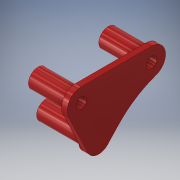
# Autodesk Inventor part: Idle pulley pin
Saved by Autodesk Inventor 2019.4 (Build 234330000, 330)
## iProperties
Created: 2020-02-23
Part Number: Idle pulley pin
Material: ABS Plastic
Document SubType Name: Modeling
Designer: admin
Density: 1.06 g/cm^3
Appearance: Red
Author: admin
Autodesk Inventor part; units mm, degrees
ref_plane "YZ Plane" through (0, 0, 0) normal (1, 0, 0) x (0, 1, 0)
ref_plane "XZ Plane" through (0, 0, 0) normal (0, 1, 0) x (-1, 0, 0)
ref_plane "XY Plane" through (0, 0, 0) normal (0, 0, 1) x (1, 0, 0)
sketch "Sketch3" plane through (0, 0, 0) normal (1, 0, 0) x (0, 1, 0)
  circle A0 centre (21.8648, -65.6605) radius 2.75 projected
  circle A1 centre (21.8648, -28.1605) radius 2.75 projected
  circle A2 centre (21.8648, 9.3395) radius 2.75 projected
  line L0 (21.8648, -65.6605) -> (21.8648, 9.3395) construction
  line L1 (29.3648, -65.6605) -> (29.3648, -28.1605) construction
  line L2 (14.3648, 9.3395) -> (14.3648, -22.1411) construction
  arc A3 (14.3648, -65.6605) -> (29.3648, -65.6605) centre (21.8648, -65.6605) ccw construction
  arc A4 (29.3648, 9.3395) -> (18.6312, 16.1066) centre (21.8648, 9.3395) ccw
  circle A5 centre (0, 0) radius 6.5
  line L3 (-2.8024, 5.8648) -> (18.6312, 16.1066)
  line L4 (-4.4137, -4.7717) -> (14.3648, -22.1411)
  arc A6 (18.6312, 16.1066) -> (14.3648, 9.3395) centre (21.8648, 9.3395) ccw
  line L5 (14.3648, -22.1411) -> (14.3648, -28.1605)
  circle A7 centre (21.8648, -28.1605) radius 7.5
  line L6 (29.3648, -28.1605) -> (29.3648, 9.3395)
  line L7 (14.3648, -28.1605) -> (14.3648, -65.6605) construction
  dimension "d14" = 15
  dimension "d15" = 13
  constraints: 21 tangent, 18 end point, 10 point on circle, 6 parallel, 5 centre point, 2 coincident, 1 midpoint, 1 vertical
  measures "d14" diameter of A4
  measures "d15" diameter of A5
extrude "Extrusion2" add sketch "Sketch3" along normal blind 3 contours L6 A7 L5 L4 A5 L3 A4 | A7 | A5
sketch "Sketch4" plane through (0, 0, 0) normal (-1, 0, 0) x (0, 0, 1)
  arc A0 (-4.7717, -4.4137) -> (5.8648, -2.8024) centre (0, 0) ccw projected
  circle A1 centre (0, 0) radius 5
  dimension "d18" = 10
  constraints: 1 centre point, 1 coincident
  measures "d18" diameter of A1
extrude "Extrusion3" add sketch "Sketch4" along normal blind 25.1
sketch "Sketch5" plane through (0, 0, 0) normal (1, 0, 0) x (0, 0, -1)
  circle A0 centre (0, 0) radius 6.5
  dimension "d23" = 13
  constraints: 1 centre point, 1 coincident
  measures "d23" diameter of A0
extrude "Extrusion4" add sketch "Sketch5" against normal blind 1.1
fillet "Fillet1" radius 50 1 edges at (1.5, 14.3648, -22.1411)
sketch "Sketch6" plane through (0, 0, 0) normal (-1, 0, 0) x (0, 0, 1)
  circle A0 centre (9.3395, 21.8648) radius 2.75 projected
  circle A1 centre (9.3395, 21.8648) radius 5
  point P0 (0, 0)
  point P1 (-65.6605, 21.8648)
  dimension "d33" = 10
  constraints: 1 centre point, 1 coincident
  measures "d33" diameter of A1
extrude "Extrusion5" add sketch "Sketch6" along normal blind 20.1
pattern_linear "Rectangular Pattern2" count 2 spacing 37.5 along (0, 0, -1) of "Extrusion5"
body "Solid2"
